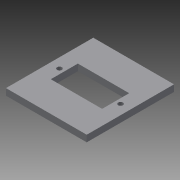
# Autodesk Inventor part: ServoHolderPlate
Saved by Autodesk Inventor 2016 (Build 200138000, 138)
## iProperties
Created: 2015-05-10
Part Number: ServoHolderPlate
Material: Generic
Document SubType Name: Modeling
Designer: Erin
Density: 1 g/cm^3
Appearance: Default
Author: Erin
Autodesk Inventor part; units mm, degrees
ref_plane "YZ Plane" through (0, 0, 0) normal (1, 0, 0) x (0, 1, 0)
ref_plane "XZ Plane" through (0, 0, 0) normal (0, 1, 0) x (-1, 0, 0)
ref_plane "XY Plane" through (0, 0, 0) normal (0, 0, 1) x (1, 0, 0)
sketch "Block1_1" plane through (0, 0, 0) normal (0, 0, 1) x (1, 0, 0)
  circle A0 centre (47.029, 24.2723) radius 1.1
  circle A1 centre (75.029, 24.2723) radius 1.1
  line L0 (49.279, 30.4723) -> (72.779, 30.4723)
  line L1 (72.779, 30.4723) -> (72.779, 18.0723)
  line L2 (72.779, 18.0723) -> (49.279, 18.0723)
  line L3 (49.279, 18.0723) -> (49.279, 30.4723)
  line L4 (49.279, 30.4723) -> (44.779, 30.4723)
  line L5 (44.779, 30.4723) -> (44.779, 18.0723)
  line L6 (44.779, 18.0723) -> (49.279, 18.0723)
  line L7 (49.279, 18.0723) -> (49.279, 30.4723)
  line L8 (72.779, 30.4723) -> (77.279, 30.4723)
  line L9 (77.279, 30.4723) -> (77.279, 18.0723)
  line L10 (77.279, 18.0723) -> (72.779, 18.0723)
  line L11 (72.779, 18.0723) -> (72.779, 30.4723)
  line L12 (44.779, 24.2723) -> (77.279, 24.2723) construction
  line L13 (61.029, 30.4723) -> (61.029, 18.0723) construction
  line L14 (47.029, 30.4723) -> (47.029, 18.0723) construction
  line L15 (75.029, 30.4723) -> (75.029, 18.0723) construction
  line L16 (66.779, 30.4723) -> (66.779, 18.0723) construction
  point P0 (60.979, 24.0984)
  dimension "d2" = 23.5
  dimension "d3" = 12.4
  dimension "d4" = 4.5
  dimension "d5" = 4.5
  dimension "d6" = 2.2
  dimension "d7" = 2.2
  dimension "d8" = 2.25
  dimension "d9" = 6
  measures "d2" distance of L1.end L2.end
  measures "d3" distance of L0.end L1.end
  measures "d4" distance of L6.end L5.end
  measures "d5" distance of L9.end L10.end
  measures "d6" diameter of A0
  measures "d7" diameter of A1
  measures "d8" distance between parallel lines of L9 L15
  measures "d9" distance between parallel lines of L16 L1
sketch "Sketch1" plane through (0, 0, 0) normal (0, 0, 1) x (1, 0, 0)
  line L0 (-18.5, 20) -> (18.5, 20)
  line L1 (18.5, 20) -> (18.5, -20)
  line L2 (18.5, -20) -> (-18.5, -20)
  line L3 (-18.5, -20) -> (-18.5, 20)
  circle A0 centre (-14, 0) radius 1.1
  circle A1 centre (14, 0) radius 1.1
  line L4 (-11.75, 6.2) -> (11.75, 6.2)
  line L5 (11.75, 6.2) -> (11.75, -6.2)
  line L6 (11.75, -6.2) -> (-11.75, -6.2)
  line L7 (-11.75, -6.2) -> (-11.75, 6.2)
  line L8 (-11.75, 6.2) -> (-16.25, 6.2)
  line L9 (-16.25, 6.2) -> (-16.25, -6.2)
  line L10 (-16.25, -6.2) -> (-11.75, -6.2)
  line L11 (-11.75, -6.2) -> (-11.75, 6.2)
  line L12 (11.75, 6.2) -> (16.25, 6.2)
  line L13 (16.25, 6.2) -> (16.25, -6.2)
  line L14 (16.25, -6.2) -> (11.75, -6.2)
  line L15 (11.75, -6.2) -> (11.75, 6.2)
  line L16 (-16.25, 0) -> (16.25, 0) construction
  line L17 (0, 6.2) -> (0, -6.2) construction
  line L18 (-14, 6.2) -> (-14, -6.2) construction
  line L19 (14, 6.2) -> (14, -6.2) construction
  line L20 (5.75, 6.2) -> (5.75, -6.2) construction
  point P0 (0, 0)
  point P1 (18.5, 0)
  point P2 (0, 20)
  point P3 (0, 0)
  dimension "d0" = 37
  dimension "d1" = 40
  constraints: 8 end point, 2 midpoint, 2 parallel, 1 coincident, 1 horizontal, 1 horizontal alignment, 1 perpendicular, 1 vertical alignment, 1 other
  measures "d0" distance of L1.end L2.end
  measures "d1" distance of L0.end L1.end
extrude "Extrusion1" add sketch "Sketch1" along normal blind 3 contours L0 L1 L2 L3 | L7 L10 L9 L8 | L12 L13 L14 L5
body "Solid1"
